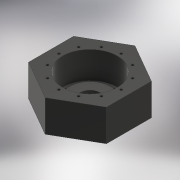
# Autodesk Inventor part: AC01
Saved by Autodesk Inventor 2017 (Build 210142000, 142)
## iProperties
Created: 2019-08-28
Part Number: AC01
Material: ABS Plastic
Document SubType Name: Modeling
Designer: Dell
Density: 1.06 g/cm^3
Appearance: Smooth - Black
Author: Dell
Autodesk Inventor part; units mm, degrees
ref_plane "YZ Plane" through (0, 0, 0) normal (1, 0, 0) x (0, 1, 0)
ref_plane "XZ Plane" through (0, 0, 0) normal (0, 1, 0) x (-1, 0, 0)
ref_plane "XY Plane" through (0, 0, 0) normal (0, 0, 1) x (1, 0, 0)
sketch "Sketch1" plane through (0, 0, 0) normal (0, 0, 1) x (1, 0, 0)
  circle A0 centre (0, 0) radius 17.5
  circle A1 centre (0, 0) radius 67.5
  circle A2 centre (41.5, 0) radius 2
  circle A3 centre (29.3449, 29.3449) radius 2
  circle A4 centre (0, 41.5) radius 2
  circle A5 centre (-29.3449, 29.3449) radius 2
  circle A6 centre (-41.5, 0) radius 2
  circle A7 centre (-29.3449, -29.3449) radius 2
  circle A8 centre (0, -41.5) radius 2
  circle A9 centre (29.3449, -29.3449) radius 2
  dimension "d0" = 35
  dimension "d1" = 135
  dimension "d2" = 4
  dimension "d3" = 41.5
  dimension "d6" = 360
  constraints: 10 centre point, 2 coincident, 1 horizontal alignment, 17 other
  measures "d0" diameter of A0
  measures "d1" diameter of A1
  measures "d2" diameter of A2
  measures "d3" distance of A2.centre point (0, 0)
extrude "Extrusion1" add sketch "Sketch1" along normal blind 15
sketch "Sketch5" plane through (0, 0, 15) normal (0, 0, 1) x (1, 0, 0)
  circle A0 centre (0, 0) radius 67.5 projected
  circle A1 centre (0, 0) radius 47.5
  dimension "d19" = 95
  constraints: 1 centre point
  measures "d19" diameter of A1
extrude "Extrusion4" add sketch "Sketch5" along normal blind 40
sketch "Sketch8" plane through (0, 0, 55) normal (0, 0, 1) x (1, 0, 0)
  circle A0 centre (-54, 0) radius 2
  circle A1 centre (-46.7654, -27) radius 2
  circle A2 centre (-27, -46.7654) radius 2
  circle A3 centre (0, -54) radius 2
  circle A4 centre (27, -46.7654) radius 2
  circle A5 centre (46.7654, -27) radius 2
  circle A6 centre (54, 0) radius 2
  circle A7 centre (46.7654, 27) radius 2
  circle A8 centre (27, 46.7654) radius 2
  circle A9 centre (0, 54) radius 2
  circle A10 centre (-27, 46.7654) radius 2
  circle A11 centre (-46.7654, 27) radius 2
  point P0 (0, 0)
  dimension "d20" = 4
  dimension "d21" = 54
  dimension "d24" = 360
  constraints: 12 centre point, 1 horizontal alignment, 25 other
  measures "d20" diameter of A0
  measures "d21" distance of point (0, 0) A0.centre
extrude "Extrusion5" cut sketch "Sketch8" against normal through all
sketch "Sketch11" plane through (0, 0, 55) normal (0, 0, 1) x (1, 0, 0)
  line L0 (0, 77.9423) -> (67.5, 38.9711)
  line L1 (67.5, 38.9711) -> (67.5, -38.9711)
  line L2 (67.5, -38.9711) -> (0, -77.9423)
  line L3 (0, -77.9423) -> (-67.5, -38.9711)
  line L4 (-67.5, -38.9711) -> (-67.5, 38.9711)
  line L5 (-67.5, 38.9711) -> (0, 77.9423)
  circle A0 centre (0, 0) radius 67.5 projected
  constraints: 12 end point, 1 coincident, 1 tangent, 1 vertical alignment, 13 other
extrude "Extrusion8" add sketch "Sketch11" against normal blind 55 contours L0 A0 L5 | L0 L1 A0 | A0 L4 L5 | L1 L2 A0 | A0 L3 L4 | L2 L3 A0
sketch "Sketch12" plane through (0, 0, 0) normal (0, 0, -1) x (-1, 0, 0)
  circle A0 centre (-54, 0) radius 2 projected
  circle A1 centre (-54, 0) radius 6.5
  circle A2 centre (-46.7654, -27) radius 6.5
  circle A3 centre (-27, -46.7654) radius 6.5
  circle A4 centre (0, -54) radius 6.5
  circle A5 centre (27, -46.7654) radius 6.5
  circle A6 centre (46.7654, -27) radius 6.5
  circle A7 centre (54, 0) radius 6.5
  circle A8 centre (46.7654, 27) radius 6.5
  circle A9 centre (27, 46.7654) radius 6.5
  circle A10 centre (0, 54) radius 6.5
  circle A11 centre (-27, 46.7654) radius 6.5
  circle A12 centre (-46.7654, 27) radius 6.5
  point P0 (0, 0)
  dimension "d37" = 13
  dimension "d40" = 360
  constraints: 12 centre point, 1 coincident, 25 other
  measures "d37" diameter of A1
extrude "Extrusion9" cut sketch "Sketch12" against normal blind 5 contours A0 | A1 | A2 | A3 | A4 | A5 | A6 | A7 | A8 | A9 | A10 | A11 | A12
sketch "Sketch16" plane through (0, 0, 15) normal (0, 0, 1) x (1, 0, 0)
  circle A0 centre (-41.5, 0) radius 2 projected
  circle A1 centre (0, 0) radius 35.5
  circle A2 centre (0, 0) radius 47.5
  line L0 (-47.5, 0) -> (-35.5, 0)
  circle A3 centre (0, 0) radius 47.5 projected
  constraints: 3 coincident, 3 horizontal alignment, 2 end point, 1 horizontal, 1 midpoint, 5 other
extrude "Extrusion11" cut sketch "Sketch16" against normal blind 7
body "Solid1"
